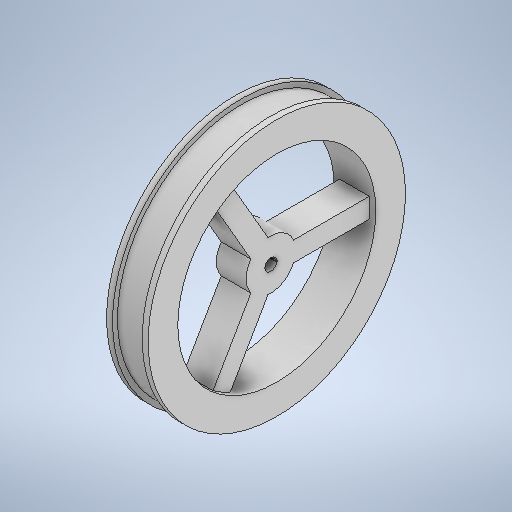
# Autodesk Inventor part: Wheel1
Saved by Autodesk Inventor 2025.2 (Build 292293000, 293)
## iProperties
Created: 2025-05-26
Part Number: Wheel1
Material: Generic
Document SubType Name: Modeling
Designer: abdal
Density: 1 g/cm^3
Appearance: Default
Author: abdal
Autodesk Inventor part; units mm, degrees
ref_plane "YZ Plane" through (0, 0, 0) normal (1, 0, 0) x (0, 1, 0)
ref_plane "XZ Plane" through (0, 0, 0) normal (0, 1, 0) x (-1, 0, 0)
sketch "Sketch1" plane through (0, 0, 0) normal (1, 0, 0) x (0, 1, 0)
  circle A0 centre (0, 0) radius 500
  circle A1 centre (0, 0) radius 625
  dimension "d0" = 1000
  dimension "d1" = 1250
  constraints: 2 centre point, 2 coincident
  measures "d0" diameter of A0
  measures "d1" diameter of A1
extrude "Extrusion1" add sketch "Sketch1" against normal blind 210
sketch "Sketch2" plane through (0, 0, 0) normal (1, 0, 0) x (0, 0, -1)
  circle A0 centre (0, 0) radius 650
  circle A1 centre (0, 0) radius 625 projected
  dimension "d4" = 1300
  constraints: 1 centre point, 1 coincident
  measures "d4" diameter of A0
sketch "Sketch3" plane through (-210, 0, 0) normal (-1, 0, 0) x (0, 0, 1)
  circle A0 centre (0, 0) radius 650
  circle A1 centre (0, 0) radius 625 projected
  dimension "d5" = 1300
  constraints: 1 centre point, 1 coincident
  measures "d5" diameter of A0
extrude "Extrusion2" add sketch "Sketch3" against normal blind 30
extrude "Extrusion3" add sketch "Sketch2" against normal blind 30
ref_plane "Work Plane1" through (-30, 0, 0) normal (1, 0, 0) x (0, 0, -1)
sketch "Sketch4" plane through (-30, 0, 0) normal (1, 0, 0) x (0, 0, -1)
  circle A0 centre (0, 0) radius 125
  dimension "d11" = 250
  constraints: 1 centre point, 1 coincident
  measures "d11" diameter of A0
extrude "Extrusion4" add sketch "Sketch4" against normal blind 150
sketch "Sketch5" plane through (-30, 0, 0) normal (1, 0, 0) x (0, 0, -1)
  line L0 (0, 0) -> (469.0204, 0) construction
  line L1 (0, 0) -> (-234.5102, 406.1836) construction
  line L2 (0, 0) -> (-234.5102, -406.1836) construction
  line L3 (0, -910) -> (0, 910) projected
  line L4 (520.2054, 50) -> (0, 50)
  line L5 (0, 50) -> (0, -50)
  line L6 (0, -50) -> (520.2054, -50)
  line L7 (520.2054, -50) -> (520.2054, 50)
  line L8 (-216.8015, 475.5111) -> (-303.404, 425.5111)
  line L9 (43.3013, 25) -> (-216.8015, 475.5111)
  line L10 (-303.404, 425.5111) -> (-43.3013, -25)
  line L11 (-43.3013, -25) -> (43.3013, 25)
  line L12 (-303.404, -425.5111) -> (-216.8015, -475.5111)
  line L13 (-43.3013, 25) -> (-303.404, -425.5111)
  line L14 (-216.8015, -475.5111) -> (43.3013, -25)
  line L15 (43.3013, -25) -> (-43.3013, 25)
  point P0 (234.5102, 0)
  point P1 (0, 0)
  point P2 (0, 0)
  point P3 (0, 0)
  point P4 (28.8675, 50)
  point P5 (-57.735, 0)
  point P6 (28.8675, -50)
  dimension "d16" = 360
  dimension "d18" = 90
  dimension "d19" = 100
  dimension "d20" = 50
  dimension "d21" = 0
  dimension "d24" = 360
  constraints: 30 end point, 2 coincident, 2 midpoint, 2 parallel, 1 horizontal, 1 perpendicular, 36 other
  measures "d18" angle of L3 L0
  measures "d19" distance between parallel lines of L4 L6
  measures "d20" distance from line of L6 point (234.51, 0)
  measures "d21" distance from line of L3 point (0, 0)
extrude "Extrusion5" add sketch "Sketch5" against normal blind 150
sketch "Sketch6" plane through (-30, 0, 0) normal (1, 0, 0) x (0, 0, -1)
  circle A0 centre (0, 0) radius 30
  dimension "d28" = 60
  constraints: 1 centre point, 1 coincident
  measures "d28" diameter of A0
extrude "Extrusion6" cut sketch "Sketch6" against normal through all
sketch "Sketch7" plane through (-30, 0, 0) normal (1, 0, 0) x (0, 0, -1)
  line L0 (33, 4) -> (28, 4)
  line L1 (28, 4) -> (28, -4)
  line L2 (28, -4) -> (33, -4)
  line L3 (33, -4) -> (33, 4)
  line L4 (910, 0) -> (-910, 0) projected
  circle A0 centre (0, 0) radius 30 projected
  point P0 (33, 0)
  dimension "d31" = 8
  dimension "d32" = 5
  dimension "d33" = 4
  dimension "d34" = 33
  constraints: 8 end point, 2 parallel, 1 horizontal, 1 midpoint, 1 perpendicular
  measures "d31" distance of L2.end L0.start
  measures "d32" distance of L1.end L2.end
  measures "d33" distance between parallel lines of L4 L2
  measures "d34" distance of A0.centre point (33, 0)
extrude "Extrusion7" cut sketch "Sketch7" against normal through all contours L3 L4 A0 L0 | A0 L4 L1 L0 | L3 L2 A0 L4 | A0 L2 L1 L4 picked at (28.627, 2.2237) picked at (28.627, -2.2237)
body "Solid1"
